Autodesk Fusion 360 part; units mm, degrees
(part 2 of 7)
  line L509 (65.8429, -65.2469) -> (65.9406, -65.3482)
  line L510 (65.9406, -65.3482) -> (66.0397, -65.448)
  line L511 (66.0397, -65.448) -> (66.1162, -65.4183)
  line L512 (66.1162, -65.4183) -> (66.1915, -65.3873)
  line L513 (66.1915, -65.3873) -> (66.2656, -65.3549)
  line L514 (66.2656, -65.3549) -> (66.3383, -65.3211)
  line L515 (66.3383, -65.3211) -> (66.4096, -65.2859)
  line L516 (66.4096, -65.2859) -> (66.4795, -65.2491)
  line L517 (66.4795, -65.2491) -> (66.5478, -65.2107)
  line L518 (66.5478, -65.2107) -> (66.6144, -65.1707)
  line L519 (66.6144, -65.1707) -> (66.6791, -65.1288)
  line L520 (66.6791, -65.1288) -> (66.7416, -65.0848)
  line L521 (66.7416, -65.0848) -> (66.8016, -65.0383)
  line L522 (66.8016, -65.0383) -> (66.8575, -64.9881)
  line L523 (66.8575, -64.9881) -> (67.1388, -64.6883)
  line L524 (67.1388, -64.6883) -> (67.2927, -64.8293)
  line L525 (67.2927, -64.8293) -> (67.4501, -64.9665)
  line L526 (67.4501, -64.9665) -> (67.6107, -65.0998)
  line L527 (67.6107, -65.0998) -> (67.7745, -65.2292)
  line L528 (67.7745, -65.2292) -> (67.5236, -65.5548)
  line L529 (67.5236, -65.5548) -> (67.483, -65.6181)
  line L530 (67.483, -65.6181) -> (67.4467, -65.6847)
  line L531 (67.4467, -65.6847) -> (67.4133, -65.7535)
  line L532 (67.4133, -65.7535) -> (67.3823, -65.8241)
  line L533 (67.3823, -65.8241) -> (67.3535, -65.8962)
  line L534 (67.3535, -65.8962) -> (67.3265, -65.9698)
  line L535 (67.3265, -65.9698) -> (67.3014, -66.0446)
  line L536 (67.3014, -66.0446) -> (67.278, -66.1207)
  line L537 (67.278, -66.1207) -> (67.2563, -66.1979)
  line L538 (67.2563, -66.1979) -> (67.2362, -66.2762)
  line L539 (67.2362, -66.2762) -> (67.2177, -66.3555)
  line L540 (67.2177, -66.3555) -> (67.2006, -66.4357)
  line L541 (67.2006, -66.4357) -> (67.315, -66.5176)
  line L542 (67.315, -66.5176) -> (67.4306, -66.5978)
  line L543 (67.4306, -66.5978) -> (67.5473, -66.6764)
  line L544 (67.5473, -66.6764) -> (67.6165, -66.6324)
  line L545 (67.6165, -66.6324) -> (67.6843, -66.5872)
  line L546 (67.6843, -66.5872) -> (67.7506, -66.541)
  line L547 (67.7506, -66.541) -> (67.8154, -66.4937)
  line L548 (67.8154, -66.4937) -> (67.8785, -66.4452)
  line L549 (67.8785, -66.4452) -> (67.9398, -66.3955)
  line L550 (67.9398, -66.3955) -> (67.9993, -66.3446)
  line L551 (67.9993, -66.3446) -> (68.0568, -66.2923)
  line L552 (68.0568, -66.2923) -> (68.1121, -66.2386)
  line L553 (68.1121, -66.2386) -> (68.1649, -66.1832)
  line L554 (68.1649, -66.1832) -> (68.2146, -66.1259)
  line L555 (68.2146, -66.1259) -> (68.2597, -66.0658)
  line L556 (68.2597, -66.0658) -> (68.477, -65.7169)
  line L557 (68.477, -65.7169) -> (68.6555, -65.8251)
  line L558 (68.6555, -65.8251) -> (68.8366, -65.929)
  line L559 (68.8366, -65.929) -> (69.0201, -66.0284)
  line L560 (69.0201, -66.0284) -> (69.206, -66.1234)
  line L561 (69.206, -66.1234) -> (69.0235, -66.4917)
  line L562 (69.0235, -66.4917) -> (68.996, -66.5617)
  line L563 (68.996, -66.5617) -> (68.9734, -66.634)
  line L564 (68.9734, -66.634) -> (68.9541, -66.708)
  line L565 (68.9541, -66.708) -> (68.9375, -66.7833)
  line L566 (68.9375, -66.7833) -> (68.9232, -66.8597)
  line L567 (68.9232, -66.8597) -> (68.9112, -66.9371)
  line L568 (68.9112, -66.9371) -> (68.9011, -67.0154)
  line L569 (68.9011, -67.0154) -> (68.8931, -67.0946)
  line L570 (68.8931, -67.0946) -> (68.8868, -67.1745)
  line L571 (68.8868, -67.1745) -> (68.8824, -67.2552)
  line L572 (68.8824, -67.2552) -> (68.8796, -67.3366)
  line L573 (68.8796, -67.3366) -> (68.8786, -67.4187)
  line L574 (68.8786, -67.4187) -> (69.0068, -67.4766)
  line L575 (69.0068, -67.4766) -> (69.1357, -67.5328)
  line L576 (69.1357, -67.5328) -> (69.2655, -67.5871)
  line L577 (69.2655, -67.5871) -> (69.3249, -67.5304)
  line L578 (69.3249, -67.5304) -> (69.3826, -67.4729)
  line L579 (69.3826, -67.4729) -> (69.4386, -67.4146)
  line L580 (69.4386, -67.4146) -> (69.4928, -67.3556)
  line L581 (69.4928, -67.3556) -> (69.5452, -67.2957)
  line L582 (69.5452, -67.2957) -> (69.5957, -67.235)
  line L583 (69.5957, -67.235) -> (69.6441, -67.1734)
  line L584 (69.6441, -67.1734) -> (69.6903, -67.1109)
  line L585 (69.6903, -67.1109) -> (69.7341, -67.0475)
  line L586 (69.7341, -67.0475) -> (69.775, -66.9829)
  line L587 (69.775, -66.9829) -> (69.8126, -66.917)
  line L588 (69.8126, -66.917) -> (69.8451, -66.8492)
  line L589 (69.8451, -66.8492) -> (69.9902, -66.4646)
  line L590 (69.9902, -66.4646) -> (70.1864, -66.5359)
  line L591 (70.1864, -66.5359) -> (70.3843, -66.6025)
  line L592 (70.3843, -66.6025) -> (70.5837, -66.6642)
  line L593 (70.5837, -66.6642) -> (70.7845, -66.7211)
  line L594 (70.7845, -66.7211) -> (70.6773, -67.1179)
  line L595 (70.6773, -67.1179) -> (70.664, -67.1919)
  line L596 (70.664, -67.1919) -> (70.656, -67.2673)
  line L597 (70.656, -67.2673) -> (70.6515, -67.3436)
  line L598 (70.6515, -67.3436) -> (70.6499, -67.4207)
  line L599 (70.6499, -67.4207) -> (70.6508, -67.4984)
  line L600 (70.6508, -67.4984) -> (70.6541, -67.5767)
  line L601 (70.6541, -67.5767) -> (70.6595, -67.6554)
  line L602 (70.6595, -67.6554) -> (70.667, -67.7347)
  line L603 (70.667, -67.7347) -> (70.6765, -67.8143)
  line L604 (70.6765, -67.8143) -> (70.6879, -67.8943)
  line L605 (70.6879, -67.8943) -> (70.7011, -67.9747)
  line L606 (70.7011, -67.9747) -> (70.7161, -68.0554)
  line L607 (70.7161, -68.0554) -> (70.8531, -68.0872)
  line L608 (70.8531, -68.0872) -> (70.9905, -68.1171)
  line L609 (70.9905, -68.1171) -> (71.1284, -68.145)
  line L610 (71.1284, -68.145) -> (71.1755, -68.0778)
  line L611 (71.1755, -68.0778) -> (71.2209, -68.0102)
  line L612 (71.2209, -68.0102) -> (71.2645, -67.9421)
  line L613 (71.2645, -67.9421) -> (71.3062, -67.8736)
  line L614 (71.3062, -67.8736) -> (71.3459, -67.8047)
  line L615 (71.3459, -67.8047) -> (71.3836, -67.7353)
  line L616 (71.3836, -67.7353) -> (71.4191, -67.6655)
  line L617 (71.4191, -67.6655) -> (71.4522, -67.5952)
  line L618 (71.4522, -67.5952) -> (71.4827, -67.5244)
  line L619 (71.4827, -67.5244) -> (71.5103, -67.4531)
  line L620 (71.5103, -67.4531) -> (71.5343, -67.3811)
  line L621 (71.5343, -67.3811) -> (71.5529, -67.3083)
  line L622 (71.5529, -67.3083) -> (71.6202, -66.9028)
  line L623 (71.6202, -66.9028) -> (71.8265, -66.9344)
  line L624 (71.8265, -66.9344) -> (72.0336, -66.9611)
  line L625 (72.0336, -66.9611) -> (72.2412, -66.9827)
  line L626 (72.2412, -66.9827) -> (72.4493, -66.9993)
  line L627 (72.4493, -66.9993) -> (72.4216, -67.4094)
  line L628 (72.4216, -67.4094) -> (72.423, -67.4846)
  line L629 (72.423, -67.4846) -> (72.4298, -67.5601)
  line L630 (72.4298, -67.5601) -> (72.4403, -67.6359)
  line L631 (72.4403, -67.6359) -> (72.4537, -67.7118)
  line L632 (72.4537, -67.7118) -> (72.4698, -67.7878)
  line L633 (72.4698, -67.7878) -> (72.4882, -67.8639)
  line L634 (72.4882, -67.8639) -> (72.509, -67.9401)
  line L635 (72.509, -67.9401) -> (72.5318, -68.0164)
  line L636 (72.5318, -68.0164) -> (72.5566, -68.0926)
  line L637 (72.5566, -68.0926) -> (72.5834, -68.1689)
  line L638 (72.5834, -68.1689) -> (72.612, -68.2451)
  line L639 (72.612, -68.2451) -> (72.6424, -68.3213)
  line L640 (72.6424, -68.3213) -> (72.783, -68.3258)
  line L641 (72.783, -68.3258) -> (72.9237, -68.3283)
  line L642 (72.9237, -68.3283) -> (73.0644, -68.3288)
  line L643 (73.0644, -68.3288) -> (73.0975, -68.2538)
  line L644 (73.0975, -68.2538) -> (73.1288, -68.1786)
  line L645 (73.1288, -68.1786) -> (73.1583, -68.1033)
  line L646 (73.1583, -68.1033) -> (73.1858, -68.028)
  line L647 (73.1858, -68.028) -> (73.2113, -67.9526)
  line L648 (73.2113, -67.9526) -> (73.2347, -67.8772)
  line L649 (73.2347, -67.8772) -> (73.2559, -67.8018)
  line L650 (73.2559, -67.8018) -> (73.2746, -67.7264)
  line L651 (73.2746, -67.7264) -> (73.2908, -67.651)
  line L652 (73.2908, -67.651) -> (73.3039, -67.5757)
  line L653 (73.3039, -67.5757) -> (73.3134, -67.5004)
  line L654 (73.3134, -67.5004) -> (73.3175, -67.4254)
  line L655 (73.3175, -67.4254) -> (73.3044, -67.0145)
  line L656 (73.3044, -67.0145) -> (73.5129, -67.0053)
  line L657 (73.5129, -67.0053) -> (73.7212, -66.9911)
  line L658 (73.7212, -66.9911) -> (73.929, -66.9718)
  line L659 (73.929, -66.9718) -> (74.1363, -66.9475)
  line L660 (74.1363, -66.9475) -> (74.1892, -67.3551)
  line L661 (74.1892, -67.3551) -> (74.2052, -67.4286)
  line L662 (74.2052, -67.4286) -> (74.2267, -67.5013)
  line L663 (74.2267, -67.5013) -> (74.2517, -67.5736)
  line L664 (74.2517, -67.5736) -> (74.2797, -67.6454)
  line L665 (74.2797, -67.6454) -> (74.3103, -67.7168)
  line L666 (74.3103, -67.7168) -> (74.3432, -67.7879)
  line L667 (74.3432, -67.7879) -> (74.3784, -67.8585)
  line L668 (74.3784, -67.8585) -> (74.4157, -67.9289)
  line L669 (74.4157, -67.9289) -> (74.4549, -67.9988)
  line L670 (74.4549, -67.9988) -> (74.496, -68.0684)
  line L671 (74.496, -68.0684) -> (74.539, -68.1376)
  line L672 (74.539, -68.1376) -> (74.5837, -68.2064)
  line L673 (74.5837, -68.2064) -> (74.7225, -68.1834)
  line L674 (74.7225, -68.1834) -> (74.8609, -68.1584)
  line L675 (74.8609, -68.1584) -> (74.999, -68.1314)
  line L676 (74.999, -68.1314) -> (75.0168, -68.0513)
  line L677 (75.0168, -68.0513) -> (75.0329, -67.9715)
  line L678 (75.0329, -67.9715) -> (75.0471, -67.8919)
  line L679 (75.0471, -67.8919) -> (75.0594, -67.8127)
  line L680 (75.0594, -67.8127) -> (75.0697, -67.7338)
  line L681 (75.0697, -67.7338) -> (75.0779, -67.6552)
  line L682 (75.0779, -67.6552) -> (75.084, -67.5771)
  line L683 (75.084, -67.5771) -> (75.0877, -67.4995)
  line L684 (75.0877, -67.4995) -> (75.0888, -67.4224)
  line L685 (75.0888, -67.4224) -> (75.087, -67.346)
  line L686 (75.087, -67.346) -> (75.0816, -67.2704)
  line L687 (75.0816, -67.2704) -> (75.071, -67.1959)
  line L688 (75.071, -67.1959) -> (74.9779, -66.7955)
  line L689 (74.9779, -66.7955) -> (75.1807, -66.7458)
  line L690 (75.1807, -66.7458) -> (75.3822, -66.6912)
  line L691 (75.3822, -66.6912) -> (75.5823, -66.6318)
  line L692 (75.5823, -66.6318) -> (75.7809, -66.5675)
  line L693 (75.7809, -66.5675) -> (75.9122, -66.957)
  line L694 (75.9122, -66.957) -> (75.9423, -67.0259)
  line L695 (75.9423, -67.0259) -> (75.9775, -67.093)
  line L696 (75.9775, -67.093) -> (76.0161, -67.159)
  line L697 (76.0161, -67.159) -> (76.0576, -67.224)
  line L698 (76.0576, -67.224) -> (76.1015, -67.2881)
  line L699 (76.1015, -67.2881) -> (76.1477, -67.3514)
  line L700 (76.1477, -67.3514) -> (76.196, -67.4138)
  line L701 (76.196, -67.4138) -> (76.2463, -67.4755)
  line L702 (76.2463, -67.4755) -> (76.2984, -67.5365)
  line L703 (76.2984, -67.5365) -> (76.3523, -67.5967)
  line L704 (76.3523, -67.5967) -> (76.4079, -67.6562)
  line L705 (76.4079, -67.6562) -> (76.4652, -67.7149)
  line L706 (76.4652, -67.7149) -> (76.5969, -67.6653)
  line L707 (76.5969, -67.6653) -> (76.7278, -67.6138)
  line L708 (76.7278, -67.6138) -> (76.8579, -67.5604)
  line L709 (76.8579, -67.5604) -> (76.8598, -67.4783)
  line L710 (76.8598, -67.4783) -> (76.8599, -67.3969)
  line L711 (76.8599, -67.3969) -> (76.8583, -67.3161)
  line L712 (76.8583, -67.3161) -> (76.8549, -67.236)
  line L713 (76.8549, -67.236) -> (76.8497, -67.1566)
  line L714 (76.8497, -67.1566) -> (76.8424, -67.0779)
  line L715 (76.8424, -67.0779) -> (76.8331, -67.0002)
  line L716 (76.8331, -67.0002) -> (76.8216, -66.9233)
  line L717 (76.8216, -66.9233) -> (76.8077, -66.8475)
  line L718 (76.8077, -66.8475) -> (76.791, -66.7729)
  line L719 (76.791, -66.7729) -> (76.771, -66.6997)
  line L720 (76.771, -66.6997) -> (76.746, -66.6288)
  line L721 (76.746, -66.6288) -> (76.5767, -66.2543)
  line L722 (76.5767, -66.2543) -> (76.7658, -66.166)
  line L723 (76.7658, -66.166) -> (76.9528, -66.0731)
  line L724 (76.9528, -66.0731) -> (77.1374, -65.9758)
  line L725 (77.1374, -65.9758) -> (77.3197, -65.8739)
  line L726 (77.3197, -65.8739) -> (77.5245, -66.2303)
  line L727 (77.5245, -66.2303) -> (77.5674, -66.2921)
  line L728 (77.5674, -66.2921) -> (77.615, -66.3511)
  line L729 (77.615, -66.3511) -> (77.6658, -66.4082)
  line L730 (77.6658, -66.4082) -> (77.7192, -66.4639)
  line L731 (77.7192, -66.4639) -> (77.7748, -66.5182)
  line L732 (77.7748, -66.5182) -> (77.8324, -66.5712)
  line L733 (77.8324, -66.5712) -> (77.892, -66.623)
  line L734 (77.892, -66.623) -> (77.9533, -66.6737)
  line L735 (77.9533, -66.6737) -> (78.0163, -66.7234)
  line L736 (78.0163, -66.7234) -> (78.0809, -66.7719)
  line L737 (78.0809, -66.7719) -> (78.1471, -66.8194)
  line L738 (78.1471, -66.8194) -> (78.2147, -66.8658)
  line L739 (78.2147, -66.8658) -> (78.3341, -66.7915)
  line L740 (78.3341, -66.7915) -> (78.4525, -66.7154)
  line L741 (78.4525, -66.7154) -> (78.5697, -66.6377)
  line L742 (78.5697, -66.6377) -> (78.5555, -66.5568)
  line L743 (78.5555, -66.5568) -> (78.5398, -66.4769)
  line L744 (78.5398, -66.4769) -> (78.5225, -66.398)
  line L745 (78.5225, -66.398) -> (78.5035, -66.3201)
  line L746 (78.5035, -66.3201) -> (78.4829, -66.2432)
  line L747 (78.4829, -66.2432) -> (78.4604, -66.1675)
  line L748 (78.4604, -66.1675) -> (78.4361, -66.093)
  line L749 (78.4361, -66.093) -> (78.4098, -66.0199)
  line L750 (78.4098, -66.0199) -> (78.3814, -65.9483)
  line L751 (78.3814, -65.9483) -> (78.3504, -65.8784)
  line L752 (78.3504, -65.8784) -> (78.3165, -65.8105)
  line L753 (78.3165, -65.8105) -> (78.2782, -65.7458)
  line L754 (78.2782, -65.7458) -> (78.0391, -65.4115)
  line L755 (78.0391, -65.4115) -> (78.2073, -65.288)
  line L756 (78.2073, -65.288) -> (78.3726, -65.1605)
  line L757 (78.3726, -65.1605) -> (78.5347, -65.0289)
  line L758 (78.5347, -65.0289) -> (78.6936, -64.8935)
  line L759 (78.6936, -64.8935) -> (78.964, -65.2031)
  line L760 (78.964, -65.2031) -> (79.0181, -65.2553)
  line L761 (79.0181, -65.2553) -> (79.0764, -65.3039)
  line L762 (79.0764, -65.3039) -> (79.1373, -65.35)
  line L763 (79.1373, -65.35) -> (79.2005, -65.3942)
  line L764 (79.2005, -65.3942) -> (79.2656, -65.4366)
  line L765 (79.2656, -65.4366) -> (79.3325, -65.4774)
  line L766 (79.3325, -65.4774) -> (79.401, -65.5166)
  line L767 (79.401, -65.5166) -> (79.4711, -65.5544)
  line L768 (79.4711, -65.5544) -> (79.5426, -65.5907)
  line L769 (79.5426, -65.5907) -> (79.6154, -65.6257)
  line L770 (79.6154, -65.6257) -> (79.6896, -65.6594)
  line L771 (79.6896, -65.6594) -> (79.765, -65.6918)
  line L772 (79.765, -65.6918) -> (79.8676, -65.5955)
  line L773 (79.8676, -65.5955) -> (79.9688, -65.4978)
  line L774 (79.9688, -65.4978) -> (80.0686, -65.3987)
  line L775 (80.0686, -65.3987) -> (80.0389, -65.3222)
  line L776 (80.0389, -65.3222) -> (80.0079, -65.2469)
  line L777 (80.0079, -65.2469) -> (79.9755, -65.1729)
  line L778 (79.9755, -65.1729) -> (79.9417, -65.1001)
  line L779 (79.9417, -65.1001) -> (79.9065, -65.0288)
  line L780 (79.9065, -65.0288) -> (79.8697, -64.9589)
  line L781 (79.8697, -64.9589) -> (79.8313, -64.8906)
  line L782 (79.8313, -64.8906) -> (79.7913, -64.824)
  line L783 (79.7913, -64.824) -> (79.7494, -64.7593)
  line L784 (79.7494, -64.7593) -> (79.7054, -64.6968)
  line L785 (79.7054, -64.6968) -> (79.6589, -64.6368)
  line L786 (79.6589, -64.6368) -> (79.6087, -64.5809)
  line L787 (79.6087, -64.5809) -> (79.3089, -64.2997)
  line L788 (79.3089, -64.2997) -> (79.4499, -64.1457)
  line L789 (79.4499, -64.1457) -> (79.5871, -63.9884)
  line L790 (79.5871, -63.9884) -> (79.7204, -63.8277)
  line L791 (79.7204, -63.8277) -> (79.8498, -63.6639)
  line L792 (79.8498, -63.6639) -> (80.1754, -63.9148)
  line L793 (80.1754, -63.9148) -> (80.2387, -63.9554)
  line L794 (80.2387, -63.9554) -> (80.3053, -63.9917)
  line L795 (80.3053, -63.9917) -> (80.3741, -64.0251)
  line L796 (80.3741, -64.0251) -> (80.4447, -64.0561)
  line L797 (80.4447, -64.0561) -> (80.5168, -64.085)
  line L798 (80.5168, -64.085) -> (80.5904, -64.1119)
  line L799 (80.5904, -64.1119) -> (80.6652, -64.137)
  line L800 (80.6652, -64.137) -> (80.7413, -64.1604)
  line L801 (80.7413, -64.1604) -> (80.8185, -64.1821)
  line L802 (80.8185, -64.1821) -> (80.8968, -64.2022)
  line L803 (80.8968, -64.2022) -> (80.9761, -64.2208)
  line L804 (80.9761, -64.2208) -> (81.0564, -64.2378)
  line L805 (81.0564, -64.2378) -> (81.1382, -64.1234)
  line L806 (81.1382, -64.1234) -> (81.2184, -64.0078)
  line L807 (81.2184, -64.0078) -> (81.297, -63.8911)
  line L808 (81.297, -63.8911) -> (81.253, -63.8219)
  line L809 (81.253, -63.8219) -> (81.2079, -63.7541)
  line L810 (81.2079, -63.7541) -> (81.1616, -63.6878)
  line L811 (81.1616, -63.6878) -> (81.1143, -63.623)
  line L812 (81.1143, -63.623) -> (81.0658, -63.56)
  line L813 (81.0658, -63.56) -> (81.0161, -63.4986)
  line L814 (81.0161, -63.4986) -> (80.9652, -63.4391)
  line L815 (80.9652, -63.4391) -> (80.9129, -63.3816)
  line L816 (80.9129, -63.3816) -> (80.8592, -63.3263)
  line L817 (80.8592, -63.3263) -> (80.8038, -63.2735)
  line L818 (80.8038, -63.2735) -> (80.7466, -63.2238)
  line L819 (80.7466, -63.2238) -> (80.6864, -63.1787)
  line L820 (80.6864, -63.1787) -> (80.3375, -62.9614)
  line L821 (80.3375, -62.9614) -> (80.4457, -62.7829)
  line L822 (80.4457, -62.7829) -> (80.5496, -62.6018)
  line L823 (80.5496, -62.6018) -> (80.649, -62.4183)
  line L824 (80.649, -62.4183) -> (80.744, -62.2324)
  line L825 (80.744, -62.2324) -> (81.1123, -62.4149)
  line L826 (81.1123, -62.4149) -> (81.1823, -62.4424)
  line L827 (81.1823, -62.4424) -> (81.2547, -62.465)
  line L828 (81.2547, -62.465) -> (81.3286, -62.4843)
  line L829 (81.3286, -62.4843) -> (81.4039, -62.501)
  line L830 (81.4039, -62.501) -> (81.4803, -62.5152)
  line L831 (81.4803, -62.5152) -> (81.5577, -62.5273)
  line L832 (81.5577, -62.5273) -> (81.636, -62.5373)
  line L833 (81.636, -62.5373) -> (81.7152, -62.5454)
  line L834 (81.7152, -62.5454) -> (81.7951, -62.5516)
  line L835 (81.7951, -62.5516) -> (81.8758, -62.5561)
  line L836 (81.8758, -62.5561) -> (81.9572, -62.5588)
  line L837 (81.9572, -62.5588) -> (82.0393, -62.5598)
  line L838 (82.0393, -62.5598) -> (82.0973, -62.4317)
  line L839 (82.0973, -62.4317) -> (82.1534, -62.3027)
  line L840 (82.1534, -62.3027) -> (82.2077, -62.1729)
  line L841 (82.2077, -62.1729) -> (82.151, -62.1136)
  line L842 (82.151, -62.1136) -> (82.0935, -62.0559)
  line L843 (82.0935, -62.0559) -> (82.0353, -61.9999)
  line L844 (82.0353, -61.9999) -> (81.9762, -61.9456)
  line L845 (81.9762, -61.9456) -> (81.9163, -61.8932)
  line L846 (81.9163, -61.8932) -> (81.8556, -61.8427)
  line L847 (81.8556, -61.8427) -> (81.794, -61.7943)
  line L848 (81.794, -61.7943) -> (81.7315, -61.7481)
  line L849 (81.7315, -61.7481) -> (81.6681, -61.7043)
  line L850 (81.6681, -61.7043) -> (81.6035, -61.6634)
  line L851 (81.6035, -61.6634) -> (81.5376, -61.6258)
  line L852 (81.5376, -61.6258) -> (81.4698, -61.5933)
  line L853 (81.4698, -61.5933) -> (81.0852, -61.4482)
  line L854 (81.0852, -61.4482) -> (81.1566, -61.252)
  line L855 (81.1566, -61.252) -> (81.2231, -61.0542)
  line L856 (81.2231, -61.0542) -> (81.2848, -60.8548)
  line L857 (81.2848, -60.8548) -> (81.3417, -60.6539)
  line L858 (81.3417, -60.6539) -> (81.7385, -60.7611)
  line L859 (81.7385, -60.7611) -> (81.8125, -60.7744)
  line L860 (81.8125, -60.7744) -> (81.8879, -60.7824)
  line L861 (81.8879, -60.7824) -> (81.9643, -60.7869)
  line L862 (81.9643, -60.7869) -> (82.0413, -60.7886)
  line L863 (82.0413, -60.7886) -> (82.119, -60.7876)
  line L864 (82.119, -60.7876) -> (82.1973, -60.7844)
  line L865 (82.1973, -60.7844) -> (82.2761, -60.7789)
  line L866 (82.2761, -60.7789) -> (82.3553, -60.7714)
  line L867 (82.3553, -60.7714) -> (82.4349, -60.7619)
  line L868 (82.4349, -60.7619) -> (82.5149, -60.7505)
  line L869 (82.5149, -60.7505) -> (82.5953, -60.7373)
  line L870 (82.5953, -60.7373) -> (82.676, -60.7224)
  line L871 (82.676, -60.7224) -> (82.7078, -60.5853)
  line L872 (82.7078, -60.5853) -> (82.7377, -60.4479)
  line L873 (82.7377, -60.4479) -> (82.7656, -60.31)
  line L874 (82.7656, -60.31) -> (82.6985, -60.2629)
  line L875 (82.6985, -60.2629) -> (82.6308, -60.2175)
  line L876 (82.6308, -60.2175) -> (82.5628, -60.1739)
  line L877 (82.5628, -60.1739) -> (82.4943, -60.1322)
  line L878 (82.4943, -60.1322) -> (82.4253, -60.0925)
  line L879 (82.4253, -60.0925) -> (82.3559, -60.0548)
  line L880 (82.3559, -60.0548) -> (82.2861, -60.0194)
  line L881 (82.2861, -60.0194) -> (82.2158, -59.9862)
  line L882 (82.2158, -59.9862) -> (82.145, -59.9557)
  line L883 (82.145, -59.9557) -> (82.0737, -59.9281)
  line L884 (82.0737, -59.9281) -> (82.0017, -59.9041)
  line L885 (82.0017, -59.9041) -> (81.9289, -59.8855)
  line L886 (81.9289, -59.8855) -> (81.5234, -59.8182)
  line L887 (81.5234, -59.8182) -> (81.5551, -59.6119)
  line L888 (81.5551, -59.6119) -> (81.5817, -59.4049)
  line L889 (81.5817, -59.4049) -> (81.6034, -59.1972)
  line L890 (81.6034, -59.1972) -> (81.6199, -58.9891)
  line L891 (81.6199, -58.9891) -> (82.0301, -59.0168)
  line L892 (82.0301, -59.0168) -> (82.1052, -59.0154)
  line L893 (82.1052, -59.0154) -> (82.1808, -59.0086)
  line L894 (82.1808, -59.0086) -> (82.2565, -58.9982)
  line L895 (82.2565, -58.9982) -> (82.3324, -58.9847)
  line L896 (82.3324, -58.9847) -> (82.4084, -58.9687)
  line L897 (82.4084, -58.9687) -> (82.4846, -58.9502)
  line L898 (82.4846, -58.9502) -> (82.5608, -58.9295)
  line L899 (82.5608, -58.9295) -> (82.637, -58.9066)
  line L900 (82.637, -58.9066) -> (82.7132, -58.8818)
  line L901 (82.7132, -58.8818) -> (82.7895, -58.855)
  line L902 (82.7895, -58.855) -> (82.8658, -58.8264)
  line L903 (82.8658, -58.8264) -> (82.942, -58.796)
  line L904 (82.942, -58.796) -> (82.9465, -58.6554)
  line L905 (82.9465, -58.6554) -> (82.949, -58.5147)
  line L906 (82.949, -58.5147) -> (82.9495, -58.374)
  line L907 (82.9495, -58.374) -> (82.8744, -58.3409)
  line L908 (82.8744, -58.3409) -> (82.7992, -58.3096)
  line L909 (82.7992, -58.3096) -> (82.7239, -58.2802)
  line L910 (82.7239, -58.2802) -> (82.6486, -58.2526)
  line L911 (82.6486, -58.2526) -> (82.5732, -58.2271)
  line L912 (82.5732, -58.2271) -> (82.4978, -58.2037)
  line L913 (82.4978, -58.2037) -> (82.4224, -58.1825)
  line L914 (82.4224, -58.1825) -> (82.347, -58.1638)
  line L915 (82.347, -58.1638) -> (82.2716, -58.1477)
  line L916 (82.2716, -58.1477) -> (82.1963, -58.1345)
  line L917 (82.1963, -58.1345) -> (82.1211, -58.125)
  line L918 (82.1211, -58.125) -> (82.046, -58.1209)
  line L919 (82.046, -58.1209) -> (81.6351, -58.1341)
  line L920 (81.6351, -58.1341) -> (81.6259, -57.9255)
  line L921 (81.6259, -57.9255) -> (81.6117, -57.7173)
  line L922 (81.6117, -57.7173) -> (81.5924, -57.5094)
  line L923 (81.5924, -57.5094) -> (81.5681, -57.3021)
  line L924 (81.5681, -57.3021) -> (81.9757, -57.2492)
  line L925 (81.9757, -57.2492) -> (82.0492, -57.2332)
  line L926 (82.0492, -57.2332) -> (82.1219, -57.2118)
  line L927 (82.1219, -57.2118) -> (82.1942, -57.1867)
  line L928 (82.1942, -57.1867) -> (82.266, -57.1588)
  line L929 (82.266, -57.1588) -> (82.3374, -57.1282)
  line L930 (82.3374, -57.1282) -> (82.4085, -57.0952)
  line L931 (82.4085, -57.0952) -> (82.4792, -57.06)
  line L932 (82.4792, -57.06) -> (82.5495, -57.0227)
  line L933 (82.5495, -57.0227) -> (82.6194, -56.9835)
  line L934 (82.6194, -56.9835) -> (82.689, -56.9424)
  line L935 (82.689, -56.9424) -> (82.7582, -56.8994)
  line L936 (82.7582, -56.8994) -> (82.827, -56.8547)
  line L937 (82.827, -56.8547) -> (82.804, -56.7159)
  line L938 (82.804, -56.7159) -> (82.779, -56.5775)
  line L939 (82.779, -56.5775) -> (82.7521, -56.4394)
  line L940 (82.7521, -56.4394) -> (82.6719, -56.4216)
  line L941 (82.6719, -56.4216) -> (82.5921, -56.4056)
  line L942 (82.5921, -56.4056) -> (82.5125, -56.3914)
  line L943 (82.5125, -56.3914) -> (82.4333, -56.3791)
  line L944 (82.4333, -56.3791) -> (82.3544, -56.3687)
  line L945 (82.3544, -56.3687) -> (82.2759, -56.3605)
  line L946 (82.2759, -56.3605) -> (82.1978, -56.3544)
  line L947 (82.1978, -56.3544) -> (82.1201, -56.3507)
  line L948 (82.1201, -56.3507) -> (82.0431, -56.3496)
  line L949 (82.0431, -56.3496) -> (81.9666, -56.3514)
  line L950 (81.9666, -56.3514) -> (81.891, -56.3568)
  line L951 (81.891, -56.3568) -> (81.8165, -56.3675)
  line L952 (81.8165, -56.3675) -> (81.4162, -56.4605)
  line L953 (81.4162, -56.4605) -> (81.3665, -56.2577)
  line L954 (81.3665, -56.2577) -> (81.3119, -56.0563)
  line L955 (81.3119, -56.0563) -> (81.2524, -55.8562)
  line L956 (81.2524, -55.8562) -> (81.1881, -55.6576)
  line L957 (81.1881, -55.6576) -> (81.5776, -55.5262)
  line L958 (81.5776, -55.5262) -> (81.6465, -55.4961)
  line L959 (81.6465, -55.4961) -> (81.7137, -55.4609)
  line L960 (81.7137, -55.4609) -> (81.7796, -55.4223)
  line L961 (81.7796, -55.4223) -> (81.8446, -55.3808)
  line L962 (81.8446, -55.3808) -> (81.9087, -55.3369)
  line L963 (81.9087, -55.3369) -> (81.972, -55.2907)
  line L964 (81.972, -55.2907) -> (82.0344, -55.2424)
  line L965 (82.0344, -55.2424) -> (82.0961, -55.1921)
  line L966 (82.0961, -55.1921) -> (82.1571, -55.14)
  line L967 (82.1571, -55.14) -> (82.2173, -55.0861)
  line L968 (82.2173, -55.0861) -> (82.2768, -55.0305)
  line L969 (82.2768, -55.0305) -> (82.3356, -54.9732)
  line L970 (82.3356, -54.9732) -> (82.2859, -54.8416)
  line L971 (82.2859, -54.8416) -> (82.2344, -54.7107)
  line L972 (82.2344, -54.7107) -> (82.181, -54.5805)
  line L973 (82.181, -54.5805) -> (82.099, -54.5786)
  line L974 (82.099, -54.5786) -> (82.0175, -54.5785)
  line L975 (82.0175, -54.5785) -> (81.9367, -54.5801)
  line L976 (81.9367, -54.5801) -> (81.8566, -54.5835)
  line L977 (81.8566, -54.5835) -> (81.7772, -54.5887)
  line L978 (81.7772, -54.5887) -> (81.6986, -54.596)
  line L979 (81.6986, -54.596) -> (81.6208, -54.6053)
  line L980 (81.6208, -54.6053) -> (81.5439, -54.6168)
  line L981 (81.5439, -54.6168) -> (81.4681, -54.6307)
  line L982 (81.4681, -54.6307) -> (81.3935, -54.6474)
  line L983 (81.3935, -54.6474) -> (81.3204, -54.6674)
  line L984 (81.3204, -54.6674) -> (81.2494, -54.6924)
  line L985 (81.2494, -54.6924) -> (80.8749, -54.8618)
  line L986 (80.8749, -54.8618) -> (80.7866, -54.6726)
  line L987 (80.7866, -54.6726) -> (80.6937, -54.4857)
  line L988 (80.6937, -54.4857) -> (80.5964, -54.301)
  line L989 (80.5964, -54.301) -> (80.4946, -54.1188)
  line L990 (80.4946, -54.1188) -> (80.851, -53.914)
  line L991 (80.851, -53.914) -> (80.9127, -53.871)
  line L992 (80.9127, -53.871) -> (80.9717, -53.8234)
  line L993 (80.9717, -53.8234) -> (81.0289, -53.7726)
  line L994 (81.0289, -53.7726) -> (81.0845, -53.7193)
  line L995 (81.0845, -53.7193) -> (81.1388, -53.6637)
  line L996 (81.1388, -53.6637) -> (81.1918, -53.606)
  line L997 (81.1918, -53.606) -> (81.2437, -53.5465)
  line L998 (81.2437, -53.5465) -> (81.2944, -53.4851)
  line L999 (81.2944, -53.4851) -> (81.344, -53.4221)
  line L1000 (81.344, -53.4221) -> (81.3925, -53.3575)
  line L1001 (81.3925, -53.3575) -> (81.44, -53.2913)
  line L1002 (81.44, -53.2913) -> (81.4865, -53.2237)
  line L1003 (81.4865, -53.2237) -> (81.4121, -53.1043)
  line L1004 (81.4121, -53.1043) -> (81.336, -52.9859)
  line L1005 (81.336, -52.9859) -> (81.2583, -52.8687)
  line L1006 (81.2583, -52.8687) -> (81.1775, -52.8829)
  line L1007 (81.1775, -52.8829) -> (81.0975, -52.8986)
  line L1008 (81.0975, -52.8986) -> (81.0186, -52.9159)
  line L1009 (81.0186, -52.9159) -> (80.9407, -52.9349)
  line L1010 (80.9407, -52.9349) -> (80.8638, -52.9556)
  line L1011 (80.8638, -52.9556) -> (80.7881, -52.978)
  line L1012 (80.7881, -52.978) -> (80.7137, -53.0023)
  line L1013 (80.7137, -53.0023) -> (80.6405, -53.0286)
  line L1014 (80.6405, -53.0286) -> (80.5689, -53.0571)
  line L1015 (80.5689, -53.0571) -> (80.499, -53.088)
  line L1016 (80.499, -53.088) -> (80.4311, -53.1219)
  line L1017 (80.4311, -53.1219) -> (80.3664, -53.1602)
  line L1018 (80.3664, -53.1602) -> (80.0321, -53.3994)
  line L1019 (80.0321, -53.3994) -> (79.9086, -53.2311)
  line L1020 (79.9086, -53.2311) -> (79.7811, -53.0658)
  line L1021 (79.7811, -53.0658) -> (79.6496, -52.9037)
  line L1022 (79.6496, -52.9037) -> (79.5142, -52.7448)
  line L1023 (79.5142, -52.7448) -> (79.8237, -52.4744)
  line L1024 (79.8237, -52.4744) -> (79.8759, -52.4203)
  line L1025 (79.8759, -52.4203) -> (79.9245, -52.3621)
  line L1026 (79.9245, -52.3621) -> (79.9707, -52.3011)
  line L1027 (79.9707, -52.3011) -> (80.0148, -52.2379)
  line L1028 (80.0148, -52.2379) -> (80.0572, -52.1728)
  line L1029 (80.0572, -52.1728) -> (80.098, -52.1059)
  line L1030 (80.098, -52.1059) -> (80.1372, -52.0374)
  line L1031 (80.1372, -52.0374) -> (80.175, -51.9673)
  line L1032 (80.175, -51.9673) -> (80.2113, -51.8959)
  line L1033 (80.2113, -51.8959) -> (80.2463, -51.823)
  line L1034 (80.2463, -51.823) -> (80.28, -51.7489)
  line L1035 (80.28, -51.7489) -> (80.3124, -51.6735)
  line L1036 (80.3124, -51.6735) -> (80.2161, -51.5709)
  line L1037 (80.2161, -51.5709) -> (80.1185, -51.4696)
  line L1038 (80.1185, -51.4696) -> (80.0193, -51.3698)
  line L1039 (80.0193, -51.3698) -> (79.9428, -51.3995)
  line L1040 (79.9428, -51.3995) -> (79.8675, -51.4305)
  line L1041 (79.8675, -51.4305) -> (79.7935, -51.4629)
  line L1042 (79.7935, -51.4629) -> (79.7207, -51.4967)
  line L1043 (79.7207, -51.4967) -> (79.6494, -51.5319)
  line L1044 (79.6494, -51.5319) -> (79.5795, -51.5687)
  line L1045 (79.5795, -51.5687) -> (79.5112, -51.6071)
  line L1046 (79.5112, -51.6071) -> (79.4446, -51.6471)
  line L1047 (79.4446, -51.6471) -> (79.3799, -51.689)
  line L1048 (79.3799, -51.689) -> (79.3174, -51.733)
  line L1049 (79.3174, -51.733) -> (79.2575, -51.7795)
  line L1050 (79.2575, -51.7795) -> (79.2015, -51.8297)
  line L1051 (79.2015, -51.8297) -> (78.9203, -52.1295)
  line L1052 (78.9203, -52.1295) -> (78.7663, -51.9885)
  line L1053 (78.7663, -51.9885) -> (78.609, -51.8513)
  line L1054 (78.609, -51.8513) -> (78.4484, -51.718)
  line L1055 (78.4484, -51.718) -> (78.2846, -51.5886)
extrude "Extrude1'" add sketch "Sketch1 (2)" along normal blind 1.7 separate body makes body 2 in component "CT idler 1"
ref_plane "WorkPlane2" through (0, 0, 38.5) normal (0, 0, 1) x (1, 0, 0) in component "CT idler 1"
sketch "Sketch2" plane through (0, 0, 38.5) normal (0, 0, 1) x (1, 0, 0) in component "CT idler 1"
  line L0 (76.1023, -58.0831) -> (76.3936, -58.0523)
  line L1 (76.3936, -58.0523) -> (76.4716, -58.0322)
  line L2 (76.4716, -58.0322) -> (76.5485, -58.0022)
  line L3 (76.5485, -58.0022) -> (76.6244, -57.9652)
  line L4 (76.6244, -57.9652) -> (76.6993, -57.9223)
  line L5 (76.6993, -57.9223) -> (76.7732, -57.8741)
  line L6 (76.7732, -57.8741) -> (76.8459, -57.8209)
  line L7 (76.8459, -57.8209) -> (76.9175, -57.7631)
  line L8 (76.9175, -57.7631) -> (76.9876, -57.7008)
  line L9 (76.9876, -57.7008) -> (77.0564, -57.6341)
  line L10 (77.0564, -57.6341) -> (77.1236, -57.5633)
  line L11 (77.1236, -57.5633) -> (77.1891, -57.4885)
  line L12 (77.1891, -57.4885) -> (77.2529, -57.4097)
  line L13 (77.2529, -57.4097) -> (77.2325, -57.3269)
  line L14 (77.2325, -57.3269) -> (77.2104, -57.2445)
  line L15 (77.2104, -57.2445) -> (77.1867, -57.1625)
  line L16 (77.1867, -57.1625) -> (77.0921, -57.1262)
  line L17 (77.0921, -57.1262) -> (76.9979, -57.0941)
  line L18 (76.9979, -57.0941) -> (76.9043, -57.0664)
  line L19 (76.9043, -57.0664) -> (76.8114, -57.0431)
  line L20 (76.8114, -57.0431) -> (76.7195, -57.0242)
  line L21 (76.7195, -57.0242) -> (76.6286, -57.0099)
  line L22 (76.6286, -57.0099) -> (76.5391, -57.0002)
  line L23 (76.5391, -57.0002) -> (76.451, -56.9954)
  line L24 (76.451, -56.9954) -> (76.3647, -56.9957)
  line L25 (76.3647, -56.9957) -> (76.2804, -57.0017)
  line L26 (76.2804, -57.0017) -> (76.1988, -57.0141)
  line L27 (76.1988, -57.0141) -> (76.1212, -57.0357)
  line L28 (76.1212, -57.0357) -> (75.8535, -57.1546)
  line L29 (75.8535, -57.1546) -> (75.7834, -57.0073)
  line L30 (75.7834, -57.0073) -> (75.7055, -56.8639)
  line L31 (75.7055, -56.8639) -> (75.6203, -56.7248)
  line L32 (75.6203, -56.7248) -> (75.5277, -56.5904)
  line L33 (75.5277, -56.5904) -> (75.7645, -56.418)
  line L34 (75.7645, -56.418) -> (75.8221, -56.3616)
  line L35 (75.8221, -56.3616) -> (75.8737, -56.2972)
  line L36 (75.8737, -56.2972) -> (75.9209, -56.2272)
  line L37 (75.9209, -56.2272) -> (75.9643, -56.1526)
  line L38 (75.9643, -56.1526) -> (76.0042, -56.0739)
  line L39 (76.0042, -56.0739) -> (76.0406, -55.9915)
  line L40 (76.0406, -55.9915) -> (76.0737, -55.9056)
  line L41 (76.0737, -55.9056) -> (76.1033, -55.8166)
  line L42 (76.1033, -55.8166) -> (76.1295, -55.7245)
  line L43 (76.1295, -55.7245) -> (76.1523, -55.6296)
  line L44 (76.1523, -55.6296) -> (76.1717, -55.532)
  line L45 (76.1717, -55.532) -> (76.1875, -55.4319)
  line L46 (76.1875, -55.4319) -> (76.1284, -55.3704)
  line L47 (76.1284, -55.3704) -> (76.0681, -55.31)
  line L48 (76.0681, -55.31) -> (76.0066, -55.2509)
  line L49 (76.0066, -55.2509) -> (75.9064, -55.2668)
  line L50 (75.9064, -55.2668) -> (75.8088, -55.2861)
  line L51 (75.8088, -55.2861) -> (75.7139, -55.3089)
  line L52 (75.7139, -55.3089) -> (75.6218, -55.3351)
  line L53 (75.6218, -55.3351) -> (75.5328, -55.3648)
  line L54 (75.5328, -55.3648) -> (75.4469, -55.3978)
  line L55 (75.4469, -55.3978) -> (75.3645, -55.4342)
  line L56 (75.3645, -55.4342) -> (75.2859, -55.4741)
  line L57 (75.2859, -55.4741) -> (75.2113, -55.5175)
  line L58 (75.2113, -55.5175) -> (75.1413, -55.5647)
  line L59 (75.1413, -55.5647) -> (75.0768, -55.6163)
  line L60 (75.0768, -55.6163) -> (75.0204, -55.6739)
  line L61 (75.0204, -55.6739) -> (74.848, -55.9107)
  line L62 (74.848, -55.9107) -> (74.7136, -55.8182)
  line L63 (74.7136, -55.8182) -> (74.5745, -55.7329)
  line L64 (74.5745, -55.7329) -> (74.4311, -55.6551)
  line L65 (74.4311, -55.6551) -> (74.2838, -55.5849)
  line L66 (74.2838, -55.5849) -> (74.4027, -55.3172)
  line L67 (74.4027, -55.3172) -> (74.4244, -55.2396)
  line L68 (74.4244, -55.2396) -> (74.4368, -55.158)
  line L69 (74.4368, -55.158) -> (74.4427, -55.0738)
  line L70 (74.4427, -55.0738) -> (74.443, -54.9874)
  line L71 (74.443, -54.9874) -> (74.4382, -54.8994)
  line L72 (74.4382, -54.8994) -> (74.4285, -54.8098)
  line L73 (74.4285, -54.8098) -> (74.4142, -54.7189)
  line L74 (74.4142, -54.7189) -> (74.3953, -54.627)
  line L75 (74.3953, -54.627) -> (74.372, -54.5341)
  line L76 (74.372, -54.5341) -> (74.3443, -54.4405)
  line L77 (74.3443, -54.4405) -> (74.3122, -54.3464)
  line L78 (74.3122, -54.3464) -> (74.2759, -54.2517)
  line L79 (74.2759, -54.2517) -> (74.1939, -54.228)
  line L80 (74.1939, -54.228) -> (74.1115, -54.2059)
  line L81 (74.1115, -54.2059) -> (74.0287, -54.1855)
  line L82 (74.0287, -54.1855) -> (73.9499, -54.2493)
  line L83 (73.9499, -54.2493) -> (73.8751, -54.3148)
  line L84 (73.8751, -54.3148) -> (73.8043, -54.382)
  line L85 (73.8043, -54.382) -> (73.7377, -54.4508)
  line L86 (73.7377, -54.4508) -> (73.6754, -54.521)
  line L87 (73.6754, -54.521) -> (73.6175, -54.5925)
  line L88 (73.6175, -54.5925) -> (73.5644, -54.6652)
  line L89 (73.5644, -54.6652) -> (73.5162, -54.7391)
  line L90 (73.5162, -54.7391) -> (73.4733, -54.814)
  line L91 (73.4733, -54.814) -> (73.4363, -54.8899)
  line L92 (73.4363, -54.8899) -> (73.4062, -54.9668)
  line L93 (73.4062, -54.9668) -> (73.3862, -55.0449)
  line L94 (73.3862, -55.0449) -> (73.3553, -55.3361)
  line L95 (73.3553, -55.3361) -> (73.1926, -55.3232)
  line L96 (73.1926, -55.3232) -> (73.0295, -55.3189)
  line L97 (73.0295, -55.3189) -> (72.8664, -55.3232)
  line L98 (72.8664, -55.3232) -> (72.7038, -55.3361)
  line L99 (72.7038, -55.3361) -> (72.6729, -55.0449)
  line L100 (72.6729, -55.0449) -> (72.6528, -54.9668)
  line L101 (72.6528, -54.9668) -> (72.6228, -54.8899)
  line L102 (72.6228, -54.8899) -> (72.5858, -54.814)
  line L103 (72.5858, -54.814) -> (72.5429, -54.7391)
  line L104 (72.5429, -54.7391) -> (72.4947, -54.6652)
  line L105 (72.4947, -54.6652) -> (72.4415, -54.5925)
  line L106 (72.4415, -54.5925) -> (72.3837, -54.521)
  line L107 (72.3837, -54.521) -> (72.3214, -54.4508)
  line L108 (72.3214, -54.4508) -> (72.2548, -54.382)
  line L109 (72.2548, -54.382) -> (72.184, -54.3148)
  line L110 (72.184, -54.3148) -> (72.1091, -54.2493)
  line L111 (72.1091, -54.2493) -> (72.0303, -54.1855)
  line L112 (72.0303, -54.1855) -> (71.9475, -54.2059)
  line L113 (71.9475, -54.2059) -> (71.8651, -54.228)
  line L114 (71.8651, -54.228) -> (71.7832, -54.2517)
  line L115 (71.7832, -54.2517) -> (71.7468, -54.3464)
  line L116 (71.7468, -54.3464) -> (71.7148, -54.4405)
  line L117 (71.7148, -54.4405) -> (71.6871, -54.5341)
  line L118 (71.6871, -54.5341) -> (71.6637, -54.627)
  line L119 (71.6637, -54.627) -> (71.6449, -54.7189)
  line L120 (71.6449, -54.7189) -> (71.6305, -54.8098)
  line L121 (71.6305, -54.8098) -> (71.6209, -54.8994)
  line L122 (71.6209, -54.8994) -> (71.6161, -54.9874)
  line L123 (71.6161, -54.9874) -> (71.6164, -55.0738)
  line L124 (71.6164, -55.0738) -> (71.6223, -55.158)
  line L125 (71.6223, -55.158) -> (71.6347, -55.2396)
  line L126 (71.6347, -55.2396) -> (71.6564, -55.3172)
  line L127 (71.6564, -55.3172) -> (71.7752, -55.5849)
  line L128 (71.7752, -55.5849) -> (71.6279, -55.6551)
  line L129 (71.6279, -55.6551) -> (71.4845, -55.7329)
  line L130 (71.4845, -55.7329) -> (71.3454, -55.8182)
  line L131 (71.3454, -55.8182) -> (71.211, -55.9107)
  line L132 (71.211, -55.9107) -> (71.0386, -55.6739)
  line L133 (71.0386, -55.6739) -> (70.9823, -55.6163)
  line L134 (70.9823, -55.6163) -> (70.9178, -55.5647)
  line L135 (70.9178, -55.5647) -> (70.8478, -55.5175)
  line L136 (70.8478, -55.5175) -> (70.7732, -55.4741)
  line L137 (70.7732, -55.4741) -> (70.6945, -55.4342)
  line L138 (70.6945, -55.4342) -> (70.6121, -55.3978)
  line L139 (70.6121, -55.3978) -> (70.5262, -55.3648)
  line L140 (70.5262, -55.3648) -> (70.4372, -55.3351)
  line L141 (70.4372, -55.3351) -> (70.3451, -55.3089)
  line L142 (70.3451, -55.3089) -> (70.2502, -55.2861)
  line L143 (70.2502, -55.2861) -> (70.1526, -55.2668)
  line L144 (70.1526, -55.2668) -> (70.0525, -55.2509)
  line L145 (70.0525, -55.2509) -> (69.991, -55.31)
  line L146 (69.991, -55.31) -> (69.9307, -55.3704)
  line L147 (69.9307, -55.3704) -> (69.8715, -55.4319)
  line L148 (69.8715, -55.4319) -> (69.8874, -55.532)
  line L149 (69.8874, -55.532) -> (69.9067, -55.6296)
  line L150 (69.9067, -55.6296) -> (69.9295, -55.7245)
  line L151 (69.9295, -55.7245) -> (69.9558, -55.8166)
  line L152 (69.9558, -55.8166) -> (69.9854, -55.9056)
  line L153 (69.9854, -55.9056) -> (70.0184, -55.9915)
  line L154 (70.0184, -55.9915) -> (70.0548, -56.0739)
  line L155 (70.0548, -56.0739) -> (70.0947, -56.1526)
  line L156 (70.0947, -56.1526) -> (70.1381, -56.2272)
  line L157 (70.1381, -56.2272) -> (70.1854, -56.2972)
  line L158 (70.1854, -56.2972) -> (70.2369, -56.3616)
  line L159 (70.2369, -56.3616) -> (70.2945, -56.418)
  line L160 (70.2945, -56.418) -> (70.5313, -56.5904)
  line L161 (70.5313, -56.5904) -> (70.4388, -56.7248)
  line L162 (70.4388, -56.7248) -> (70.3535, -56.8639)
  line L163 (70.3535, -56.8639) -> (70.2757, -57.0073)
  line L164 (70.2757, -57.0073) -> (70.2055, -57.1546)
  line L165 (70.2055, -57.1546) -> (69.9379, -57.0357)
  line L166 (69.9379, -57.0357) -> (69.8602, -57.0141)
  line L167 (69.8602, -57.0141) -> (69.7786, -57.0017)
  line L168 (69.7786, -57.0017) -> (69.6944, -56.9957)
  line L169 (69.6944, -56.9957) -> (69.6081, -56.9954)
  line L170 (69.6081, -56.9954) -> (69.52, -57.0002)
  line L171 (69.52, -57.0002) -> (69.4304, -57.0099)
  line L172 (69.4304, -57.0099) -> (69.3396, -57.0242)
  line L173 (69.3396, -57.0242) -> (69.2476, -57.0431)
  line L174 (69.2476, -57.0431) -> (69.1548, -57.0664)
  line L175 (69.1548, -57.0664) -> (69.0612, -57.0941)
  line L176 (69.0612, -57.0941) -> (68.967, -57.1262)
  line L177 (68.967, -57.1262) -> (68.8723, -57.1625)
  line L178 (68.8723, -57.1625) -> (68.8486, -57.2445)
  line L179 (68.8486, -57.2445) -> (68.8266, -57.3269)
  line L180 (68.8266, -57.3269) -> (68.8061, -57.4097)
  line L181 (68.8061, -57.4097) -> (68.8699, -57.4885)
  line L182 (68.8699, -57.4885) -> (68.9354, -57.5633)
  line L183 (68.9354, -57.5633) -> (69.0027, -57.6341)
  line L184 (69.0027, -57.6341) -> (69.0714, -57.7008)
  line L185 (69.0714, -57.7008) -> (69.1416, -57.7631)
  line L186 (69.1416, -57.7631) -> (69.2131, -57.8209)
  line L187 (69.2131, -57.8209) -> (69.2858, -57.8741)
  line L188 (69.2858, -57.8741) -> (69.3597, -57.9223)
  line L189 (69.3597, -57.9223) -> (69.4346, -57.9652)
  line L190 (69.4346, -57.9652) -> (69.5105, -58.0022)
  line L191 (69.5105, -58.0022) -> (69.5874, -58.0322)
  line L192 (69.5874, -58.0322) -> (69.6655, -58.0523)
  line L193 (69.6655, -58.0523) -> (69.9567, -58.0831)
  line L194 (69.9567, -58.0831) -> (69.9438, -58.2458)
  line L195 (69.9438, -58.2458) -> (69.9395, -58.4089)
  line L196 (69.9395, -58.4089) -> (69.9438, -58.572)
  line L197 (69.9438, -58.572) -> (69.9567, -58.7347)
  line L198 (69.9567, -58.7347) -> (69.6655, -58.7655)
  line L199 (69.6655, -58.7655) -> (69.5874, -58.7856)
  line L200 (69.5874, -58.7856) -> (69.5105, -58.8156)
  line L201 (69.5105, -58.8156) -> (69.4346, -58.8526)
  line L202 (69.4346, -58.8526) -> (69.3597, -58.8955)
  line L203 (69.3597, -58.8955) -> (69.2858, -58.9437)
  line L204 (69.2858, -58.9437) -> (69.2131, -58.9969)
  line L205 (69.2131, -58.9969) -> (69.1416, -59.0547)
  line L206 (69.1416, -59.0547) -> (69.0714, -59.117)
  line L207 (69.0714, -59.117) -> (69.0027, -59.1837)
  line L208 (69.0027, -59.1837) -> (68.9354, -59.2545)
  line L209 (68.9354, -59.2545) -> (68.8699, -59.3293)
  line L210 (68.8699, -59.3293) -> (68.8061, -59.4081)
  line L211 (68.8061, -59.4081) -> (68.8266, -59.4909)
  line L212 (68.8266, -59.4909) -> (68.8486, -59.5733)
  line L213 (68.8486, -59.5733) -> (68.8723, -59.6553)
  line L214 (68.8723, -59.6553) -> (68.967, -59.6916)
  line L215 (68.967, -59.6916) -> (69.0612, -59.7237)
  line L216 (69.0612, -59.7237) -> (69.1548, -59.7514)
  line L217 (69.1548, -59.7514) -> (69.2476, -59.7747)
  line L218 (69.2476, -59.7747) -> (69.3396, -59.7936)
  line L219 (69.3396, -59.7936) -> (69.4304, -59.8079)
  line L220 (69.4304, -59.8079) -> (69.52, -59.8175)
  line L221 (69.52, -59.8175) -> (69.6081, -59.8224)
  line L222 (69.6081, -59.8224) -> (69.6944, -59.822)
  line L223 (69.6944, -59.822) -> (69.7786, -59.8161)
  line L224 (69.7786, -59.8161) -> (69.8602, -59.8037)
  line L225 (69.8602, -59.8037) -> (69.9379, -59.7821)
  line L226 (69.9379, -59.7821) -> (70.2055, -59.6632)
  line L227 (70.2055, -59.6632) -> (70.2757, -59.8105)
  line L228 (70.2757, -59.8105) -> (70.3535, -59.9539)
  line L229 (70.3535, -59.9539) -> (70.4388, -60.093)
  line L230 (70.4388, -60.093) -> (70.5313, -60.2274)
  line L231 (70.5313, -60.2274) -> (70.2945, -60.3998)
  line L232 (70.2945, -60.3998) -> (70.2369, -60.4562)
  line L233 (70.2369, -60.4562) -> (70.1854, -60.5206)
  line L234 (70.1854, -60.5206) -> (70.1381, -60.5906)
  line L235 (70.1381, -60.5906) -> (70.0947, -60.6652)
  line L236 (70.0947, -60.6652) -> (70.0548, -60.7439)
  line L237 (70.0548, -60.7439) -> (70.0184, -60.8263)
  line L238 (70.0184, -60.8263) -> (69.9854, -60.9122)
  line L239 (69.9854, -60.9122) -> (69.9558, -61.0012)
  line L240 (69.9558, -61.0012) -> (69.9295, -61.0933)
  line L241 (69.9295, -61.0933) -> (69.9067, -61.1882)
  line L242 (69.9067, -61.1882) -> (69.8874, -61.2858)
  line L243 (69.8874, -61.2858) -> (69.8715, -61.3859)
  line L244 (69.8715, -61.3859) -> (69.9307, -61.4474)
  line L245 (69.9307, -61.4474) -> (69.991, -61.5078)
  line L246 (69.991, -61.5078) -> (70.0525, -61.5669)
  line L247 (70.0525, -61.5669) -> (70.1526, -61.551)
  line L248 (70.1526, -61.551) -> (70.2502, -61.5317)
  line L249 (70.2502, -61.5317) -> (70.3451, -61.5089)
  line L250 (70.3451, -61.5089) -> (70.4372, -61.4827)
  line L251 (70.4372, -61.4827) -> (70.5262, -61.453)
  line L252 (70.5262, -61.453) -> (70.6121, -61.42)
  line L253 (70.6121, -61.42) -> (70.6945, -61.3836)
  line L254 (70.6945, -61.3836) -> (70.7732, -61.3437)
  line L255 (70.7732, -61.3437) -> (70.8478, -61.3003)
  line L256 (70.8478, -61.3003) -> (70.9178, -61.2531)
  line L257 (70.9178, -61.2531) -> (70.9823, -61.2015)
  line L258 (70.9823, -61.2015) -> (71.0386, -61.1439)
  line L259 (71.0386, -61.1439) -> (71.211, -60.9071)
  line L260 (71.211, -60.9071) -> (71.3454, -60.9996)
  line L261 (71.3454, -60.9996) -> (71.4845, -61.0849)
  line L262 (71.4845, -61.0849) -> (71.6279, -61.1627)
  line L263 (71.6279, -61.1627) -> (71.7752, -61.2329)
  line L264 (71.7752, -61.2329) -> (71.6564, -61.5006)
  line L265 (71.6564, -61.5006) -> (71.6347, -61.5782)
  line L266 (71.6347, -61.5782) -> (71.6223, -61.6598)
  line L267 (71.6223, -61.6598) -> (71.6164, -61.744)
  line L268 (71.6164, -61.744) -> (71.6161, -61.8304)
  line L269 (71.6161, -61.8304) -> (71.6209, -61.9184)
  line L270 (71.6209, -61.9184) -> (71.6305, -62.008)
  line L271 (71.6305, -62.008) -> (71.6449, -62.0989)
  line L272 (71.6449, -62.0989) -> (71.6637, -62.1908)
  line L273 (71.6637, -62.1908) -> (71.6871, -62.2837)
  line L274 (71.6871, -62.2837) -> (71.7148, -62.3773)
  line L275 (71.7148, -62.3773) -> (71.7468, -62.4714)
  line L276 (71.7468, -62.4714) -> (71.7832, -62.5661)
  line L277 (71.7832, -62.5661) -> (71.8651, -62.5898)
  line L278 (71.8651, -62.5898) -> (71.9475, -62.6119)
  line L279 (71.9475, -62.6119) -> (72.0303, -62.6323)
  line L280 (72.0303, -62.6323) -> (72.1091, -62.5685)
  line L281 (72.1091, -62.5685) -> (72.184, -62.503)
  line L282 (72.184, -62.503) -> (72.2548, -62.4358)
  line L283 (72.2548, -62.4358) -> (72.3214, -62.367)
  line L284 (72.3214, -62.367) -> (72.3837, -62.2968)
  line L285 (72.3837, -62.2968) -> (72.4415, -62.2253)
  line L286 (72.4415, -62.2253) -> (72.4947, -62.1526)
  line L287 (72.4947, -62.1526) -> (72.5429, -62.0787)
  line L288 (72.5429, -62.0787) -> (72.5858, -62.0038)
  line L289 (72.5858, -62.0038) -> (72.6228, -61.9279)
  line L290 (72.6228, -61.9279) -> (72.6528, -61.851)
  line L291 (72.6528, -61.851) -> (72.6729, -61.7729)
  line L292 (72.6729, -61.7729) -> (72.7038, -61.4817)
  line L293 (72.7038, -61.4817) -> (72.8664, -61.4946)
  line L294 (72.8664, -61.4946) -> (73.0295, -61.4989)
  line L295 (73.0295, -61.4989) -> (73.1926, -61.4946)
  line L296 (73.1926, -61.4946) -> (73.3553, -61.4817)
  line L297 (73.3553, -61.4817) -> (73.3862, -61.7729)
  line L298 (73.3862, -61.7729) -> (73.4062, -61.851)
  line L299 (73.4062, -61.851) -> (73.4363, -61.9279)
  line L300 (73.4363, -61.9279) -> (73.4733, -62.0038)
  line L301 (73.4733, -62.0038) -> (73.5162, -62.0787)
  line L302 (73.5162, -62.0787) -> (73.5644, -62.1526)
  line L303 (73.5644, -62.1526) -> (73.6175, -62.2253)
  line L304 (73.6175, -62.2253) -> (73.6754, -62.2968)
  line L305 (73.6754, -62.2968) -> (73.7377, -62.367)
  line L306 (73.7377, -62.367) -> (73.8043, -62.4358)
  line L307 (73.8043, -62.4358) -> (73.8751, -62.503)
  line L308 (73.8751, -62.503) -> (73.9499, -62.5685)
  line L309 (73.9499, -62.5685) -> (74.0287, -62.6323)
  line L310 (74.0287, -62.6323) -> (74.1115, -62.6119)
  line L311 (74.1115, -62.6119) -> (74.1939, -62.5898)
  line L312 (74.1939, -62.5898) -> (74.2759, -62.5661)
  line L313 (74.2759, -62.5661) -> (74.3122, -62.4714)
  line L314 (74.3122, -62.4714) -> (74.3443, -62.3773)
  line L315 (74.3443, -62.3773) -> (74.372, -62.2837)
  line L316 (74.372, -62.2837) -> (74.3953, -62.1908)
  line L317 (74.3953, -62.1908) -> (74.4142, -62.0989)
  line L318 (74.4142, -62.0989) -> (74.4285, -62.008)
  line L319 (74.4285, -62.008) -> (74.4382, -61.9184)
  line L320 (74.4382, -61.9184) -> (74.443, -61.8304)
  line L321 (74.443, -61.8304) -> (74.4427, -61.744)
  line L322 (74.4427, -61.744) -> (74.4368, -61.6598)
  line L323 (74.4368, -61.6598) -> (74.4244, -61.5782)
  line L324 (74.4244, -61.5782) -> (74.4027, -61.5006)
  line L325 (74.4027, -61.5006) -> (74.2838, -61.2329)
  line L326 (74.2838, -61.2329) -> (74.4311, -61.1627)
  line L327 (74.4311, -61.1627) -> (74.5745, -61.0849)
  line L328 (74.5745, -61.0849) -> (74.7136, -60.9996)
  line L329 (74.7136, -60.9996) -> (74.848, -60.9071)
  line L330 (74.848, -60.9071) -> (75.0204, -61.1439)
  line L331 (75.0204, -61.1439) -> (75.0768, -61.2015)
  line L332 (75.0768, -61.2015) -> (75.1413, -61.2531)
  line L333 (75.1413, -61.2531) -> (75.2113, -61.3003)
  line L334 (75.2113, -61.3003) -> (75.2859, -61.3437)
  line L335 (75.2859, -61.3437) -> (75.3645, -61.3836)
  line L336 (75.3645, -61.3836) -> (75.4469, -61.42)
  line L337 (75.4469, -61.42) -> (75.5328, -61.453)
  line L338 (75.5328, -61.453) -> (75.6218, -61.4827)
  line L339 (75.6218, -61.4827) -> (75.7139, -61.5089)
  line L340 (75.7139, -61.5089) -> (75.8088, -61.5317)
  line L341 (75.8088, -61.5317) -> (75.9064, -61.551)
  line L342 (75.9064, -61.551) -> (76.0066, -61.5669)
  line L343 (76.0066, -61.5669) -> (76.0681, -61.5078)
  line L344 (76.0681, -61.5078) -> (76.1284, -61.4474)
  line L345 (76.1284, -61.4474) -> (76.1875, -61.3859)
  line L346 (76.1875, -61.3859) -> (76.1717, -61.2858)
  line L347 (76.1717, -61.2858) -> (76.1523, -61.1882)
  line L348 (76.1523, -61.1882) -> (76.1295, -61.0933)
  line L349 (76.1295, -61.0933) -> (76.1033, -61.0012)
  line L350 (76.1033, -61.0012) -> (76.0737, -60.9122)
  line L351 (76.0737, -60.9122) -> (76.0406, -60.8263)
  line L352 (76.0406, -60.8263) -> (76.0042, -60.7439)
  line L353 (76.0042, -60.7439) -> (75.9643, -60.6652)
  line L354 (75.9643, -60.6652) -> (75.9209, -60.5906)
  line L355 (75.9209, -60.5906) -> (75.8737, -60.5206)
  line L356 (75.8737, -60.5206) -> (75.8221, -60.4562)
  line L357 (75.8221, -60.4562) -> (75.7645, -60.3998)
  line L358 (75.7645, -60.3998) -> (75.5277, -60.2274)
  line L359 (75.5277, -60.2274) -> (75.6203, -60.093)
  line L360 (75.6203, -60.093) -> (75.7055, -59.9539)
  line L361 (75.7055, -59.9539) -> (75.7834, -59.8105)